Autodesk Fusion 360 part; units mm, degrees
(part 4 of 5)
  constraint parallel L69 L71
  constraint tangent L69 A64
  constraint tangent L72 A64
  constraint tangent L71 A65
  constraint tangent L72 A65
  constraint tangent L70 A66
  constraint tangent L71 A66
  constraint tangent L69 A67
  constraint tangent L70 A67
  constraint tangent L73 A68
  constraint tangent L76 A68
  constraint tangent L75 A69
  constraint tangent L76 A69
  constraint tangent L74 A70
  constraint tangent L75 A70
  constraint tangent L73 A71
  constraint tangent L74 A71
  constraint tangent L79 A72
  constraint tangent L77 A73
  constraint equal A72 A73
  constraint tangent L77 A74
  constraint tangent L78 A74
  constraint tangent L78 A75
  constraint tangent L79 A75
  constraint tangent L84 A76
  constraint tangent L85 A76
  constraint tangent L85 A77
  constraint tangent L86 A77
  constraint tangent L86 A78
  constraint tangent L87 A78
  constraint tangent L84 A79
  constraint tangent L87 A79
  constraint tangent L82 A80
  constraint tangent L83 A80
  constraint tangent L81 A81
  constraint tangent L82 A81
  constraint tangent L80 A82
  constraint tangent L81 A82
  constraint tangent L80 A83
  constraint tangent L83 A83
  constraint vertical L86
  constraint parallel L79 L86
  constraint coincident A72.start A73.end
  measures "d463" radius of A0
  measures "d464" radius of A2
  measures "d465" radius of A3
  measures "d466" radius of A6
  measures "d467" radius of A7
  measures "d468" radius of A8
  measures "d469" radius of A9
  measures "d470" radius of A10
  measures "d471" radius of A11
  measures "d472" radius of A12
  measures "d473" radius of A13
  measures "d474" radius of A14
  measures "d475" radius of A15
  measures "d476" radius of A16
  measures "d477" radius of A17
  measures "d478" radius of A18
  measures "d479" radius of A19
  measures "d480" radius of A20
  measures "d481" radius of A21
  measures "d482" radius of A22
  measures "d483" radius of A23
  measures "d484" radius of A24
  measures "d485" radius of A25
  measures "d486" radius of A26
  measures "d487" radius of A27
  measures "d488" radius of A28
  measures "d489" radius of A29
  measures "d490" radius of A30
  measures "d491" radius of A31
  measures "d492" radius of A32
  measures "d493" radius of A33
  measures "d494" radius of A34
  measures "d495" radius of A35
  measures "d496" radius of A36
  measures "d497" radius of A37
  measures "d498" radius of A38
  measures "d499" radius of A39
  measures "d500" radius of A40
  measures "d501" radius of A41
  measures "d502" radius of A42
  measures "d503" radius of A43
  measures "d504" radius of A45
  measures "d505" radius of A46
  measures "d506" radius of A47
  measures "d507" radius of A48
  measures "d508" radius of A49
  measures "d509" radius of A50
  measures "d510" radius of A51
  measures "d511" radius of A52
  measures "d512" radius of A53
  measures "d513" radius of A54
  measures "d514" radius of A55
  measures "d515" radius of A56
  measures "d516" radius of A57
  measures "d517" radius of A58
  measures "d518" radius of A59
  measures "d519" radius of A60
  measures "d520" radius of A61
  measures "d521" radius of A63
  measures "d522" radius of A64
  measures "d523" radius of A65
  measures "d524" radius of A66
  measures "d525" radius of A67
  measures "d526" radius of A68
  measures "d527" radius of A69
  measures "d528" radius of A70
  measures "d529" radius of A71
  measures "d530" radius of A72
  measures "d531" radius of A74
  measures "d532" radius of A75
  measures "d533" radius of A76
  measures "d534" radius of A77
  measures "d535" radius of A78
  measures "d536" radius of A79
  measures "d537" radius of A80
  measures "d538" radius of A81
  measures "d539" radius of A82
  measures "d540" radius of A83
extrude "Extrude10" cut sketch "Sketch22" along normal up to surface contours L7 L8 L9 A3 A4 A5 | L10 L11 L12 A6 A7 A8 | L14 L15 L16 L17 A9 A10 A11 A12 | L18 L19 L20 L21 A13 A14 A15 A16 | L23 L24 L25 L26 A17 A18 A19 A20 | L27 L28 L29 L30 A21 A22 A23 A24 | L31 L32 L33 A25 A26 A27 A28 | L34 L35 L36 A29 A30 A31 | L37 L38 L39 L40 A32 A33 A34 A35 | L41 L42 L43 A36 A37 A38 | L44 L45 L46 L47 A39 A40 A41 A42 | L48 L49 L50 A43 A44 A45 | L51 L52 L53 A46 A47 A48 | L54 L55 L56 L57 A49 A50 A51 A52 | L58 L59 L60 A53 A54 A55 | L61 L62 L63 L64 A56 A57 A58 A59 | L65 L66 L67 L68 A60 A61 A62 A63 | L69 L70 L72 A64 A65 A66 A67 | L73 L74 L75 L76 A68 A69 A70 A71 | L80 L81 L82 L83 A80 A81 A82 A83 | L84 L85 L86 L87 A76 A77 A78 A79 end surface through (-10.2751, 292.6499, 24.2874) normal (-0.992191, 0, 0.12473) offset 0
extrude "Extrude11" cut sketch "Sketch22" against normal blind 3 contours L4 L5 L6 A0 A1 A2 | L77 L78 L79 A72 A73 A74 A75
sketch "Sketch23" plane through (-113.7873, 0, 0) normal (-1, 0, 0) x (0, -1, 0)
  line L0 (-298.2923, 37.3) -> (-298, 21.0097)
  line L1 (-298, 21.0097) -> (-298.5325, 4.9975)
  line L2 (-298.5325, 4.9975) -> (-2.7182, 4.9975)
  line L3 (-2.9579, 37.3) -> (-298.2923, 37.3)
  line L4 (-3.7376, 32.7885) -> (-2.7977, 24.3512)
  line L5 (-3.3467, 19.0615) -> (-6.362, 9.8946)
  line L6 (-9.6868, 7.4883) -> (-12.9772, 7.4883)
  line L7 (-15.4767, 9.9351) -> (-15.9653, 32.9032)
  line L8 (-13.4659, 35.4563) -> (-6.7191, 35.4563)
  arc A0 (-3.7376, 32.7885) -> (-6.7191, 35.4563) centre (-6.7191, 32.4563) ccw
  arc A1 (-3.3467, 19.0615) -> (-2.7977, 24.3512) centre (-15.2208, 22.9673) ccw
  arc A2 (-9.6868, 7.4883) -> (-6.362, 9.8946) centre (-9.6868, 10.9883) ccw
  arc A3 (-15.4767, 9.9351) -> (-12.9772, 7.4883) centre (-12.9772, 9.9883) ccw
  arc A4 (-13.4659, 35.4563) -> (-15.9653, 32.9032) centre (-13.4659, 32.9563) ccw
  line L9 (-29.0847, 30.6184) -> (-17.0847, 30.6184)
  line L10 (-13.0847, 26.6184) -> (-13.0847, 14.6184)
  line L11 (-17.0847, 10.6184) -> (-29.0847, 10.6184)
  line L12 (-33.0847, 14.6184) -> (-33.0847, 26.6184)
  arc A5 (-33.0847, 14.6184) -> (-29.0847, 10.6184) centre (-29.0847, 14.6184) ccw
  arc A6 (-13.0847, 26.6184) -> (-17.0847, 30.6184) centre (-17.0847, 26.6184) ccw
  arc A7 (-17.0847, 10.6184) -> (-13.0847, 14.6184) centre (-17.0847, 14.6184) ccw
  arc A8 (-29.0847, 30.6184) -> (-33.0847, 26.6184) centre (-29.0847, 26.6184) ccw
  line L13 (-18.1072, 11.7154) -> (-18.1072, 8.9883)
  line L14 (-19.6072, 7.4883) -> (-30.6835, 7.4883)
  line L15 (-32.5016, 8.6549) -> (-32.5191, 8.693)
  line L16 (-32.0267, 10.0187) -> (-28.3251, 11.7154)
  line L17 (-28.3251, 11.7154) -> (-18.1072, 11.7154)
  arc A9 (-19.6072, 7.4883) -> (-18.1072, 8.9883) centre (-19.6072, 8.9883) ccw
  arc A10 (-32.5016, 8.6549) -> (-30.6835, 7.4883) centre (-30.6835, 9.4883) ccw
  arc A11 (-32.0267, 10.0187) -> (-32.5191, 8.693) centre (-31.61, 9.1097) ccw
  line L18 (-50.0683, 30.66) -> (-37.8488, 14.315)
  line L19 (-33.932, 14.2042) -> (-18.1542, 32.9917)
  line L20 (-19.3029, 35.4563) -> (-47.6655, 35.4563)
  arc A12 (-18.1542, 32.9917) -> (-19.3029, 35.4563) centre (-19.3029, 33.9563) ccw
  arc A13 (-47.6655, 35.4563) -> (-50.0683, 30.66) centre (-47.6655, 32.4563) ccw
  arc A14 (-37.8488, 14.315) -> (-33.932, 14.2042) centre (-35.8465, 15.812) ccw
  line L21 (-80.2589, 32.3275) -> (-72.3955, 20.8271)
  line L22 (-67.1338, 20.2294) -> (-53.4418, 32.8535)
  line L23 (-54.4585, 35.4563) -> (-78.6079, 35.4563)
  arc A15 (-53.4418, 32.8535) -> (-54.4585, 35.4563) centre (-54.4585, 33.9563) ccw
  arc A16 (-72.3955, 20.8271) -> (-67.1338, 20.2294) centre (-69.5063, 22.8025) ccw
  arc A17 (-78.6079, 35.4563) -> (-80.2589, 32.3275) centre (-78.6079, 33.4563) ccw
  line L24 (-50.8537, 28.3512) -> (-36.6087, 9.9051)
  line L25 (-37.7959, 7.4883) -> (-71.2302, 7.4883)
  line L26 (-61.4756, 22.7149) -> (-55.3137, 28.674)
  arc A18 (-50.8537, 28.3512) -> (-55.3137, 28.674) centre (-53.2281, 26.5175) ccw
  arc A19 (-37.7959, 7.4883) -> (-36.6087, 9.9051) centre (-37.7959, 8.9883) ccw
  arc A20 (-72.4665, 9.8377) -> (-71.2302, 7.4883) centre (-71.2302, 8.9883) ccw
  arc A21 (-61.4756, 22.7149) -> (-72.5137, 9.7645) centre (0.0474, -40.9024) ccw
  line L27 (-82.205, 31.3656) -> (-72.5578, 17.4373)
  line L28 (-72.8035, 13.7118) -> (-73.5988, 12.8364)
  line L29 (-78.0703, 11.8224) -> (-104.2986, 22.522)
  line L30 (-105.4935, 24.8169) -> (-103.8723, 31.9532)
  line L31 (-99.4841, 35.4563) -> (-90.0147, 35.4563)
  arc A22 (-78.0703, 11.8224) -> (-73.5988, 12.8364) centre (-76.5594, 15.5261) ccw
  arc A23 (-72.8035, 13.7118) -> (-72.5578, 17.4373) centre (-75.024, 15.7291) ccw
  arc A24 (-82.205, 31.3656) -> (-90.0147, 35.4563) centre (-90.0147, 25.9563) ccw
  arc A25 (-99.4841, 35.4563) -> (-103.8723, 31.9532) centre (-99.4841, 30.9563) ccw
  arc A26 (-105.4935, 24.8169) -> (-104.2986, 22.522) centre (-103.5432, 24.3738) ccw
  line L32 (-102.0259, 19.6707) -> (-78.925, 9.4021)
  line L33 (-79.3311, 7.4883) -> (-116.1348, 7.4883)
  line L34 (-117.4703, 10.977) -> (-109.0066, 18.5695)
  arc A27 (-102.0259, 19.6707) -> (-109.0066, 18.5695) centre (-104.6662, 13.7311) ccw
  arc A28 (-79.3311, 7.4883) -> (-78.925, 9.4021) centre (-79.3311, 8.4883) ccw
  arc A29 (-117.4703, 10.977) -> (-116.1348, 7.4883) centre (-116.1348, 9.4883) ccw
  line L35 (-127.6369, 31.7266) -> (-123.0407, 13.3976)
  line L36 (-118.0109, 12.0045) -> (-109.066, 20.9374)
  line L37 (-106.5273, 25.9576) -> (-105.6108, 32.007)
  line L38 (-108.577, 35.4563) -> (-124.727, 35.4563)
  arc A30 (-105.6108, 32.007) -> (-108.577, 35.4563) centre (-108.577, 32.4563) ccw
  arc A31 (-109.066, 20.9374) -> (-106.5273, 25.9576) centre (-115.4257, 27.3056) ccw
  arc A32 (-123.0407, 13.3976) -> (-118.0109, 12.0045) centre (-120.1308, 14.1272) ccw
  arc A33 (-124.727, 35.4563) -> (-127.6369, 31.7266) centre (-124.727, 32.4563) ccw
  line L39 (-130.3627, 33.6384) -> (-123.8711, 10.6682)
  line L40 (-126.2769, 7.4883) -> (-169.5459, 7.4883)
  line L41 (-170.2607, 9.1876) -> (-147.4375, 32.5152)
  line L42 (-139.5747, 35.8225) -> (-133.2496, 35.8225)
  arc A34 (-130.3627, 33.6384) -> (-133.2496, 35.8225) centre (-133.2496, 32.8225) ccw
  arc A35 (-139.5747, 35.8225) -> (-147.4375, 32.5152) centre (-139.5747, 24.8225) ccw
  arc A36 (-126.2769, 7.4883) -> (-123.8711, 10.6682) centre (-126.2769, 9.9883) ccw
  arc A37 (-170.2607, 9.1876) -> (-169.5459, 7.4883) centre (-169.5459, 8.4883) ccw
  line L43 (-171.6146, 10.8227) -> (-150.4805, 32.4238)
  line L44 (-151.9101, 35.8225) -> (-177.6214, 35.8225)
  line L45 (-181.99, 32.4024) -> (-182.3695, 30.8671)
  line L46 (-181.8959, 26.7134) -> (-174.0246, 11.1932)
  arc A38 (-182.3695, 30.8671) -> (-181.8959, 26.7134) centre (-176.5448, 29.4273) ccw
  arc A39 (-177.6214, 35.8225) -> (-181.99, 32.4024) centre (-177.6214, 31.3225) ccw
  arc A40 (-174.0246, 11.1932) -> (-171.6146, 10.8227) centre (-172.6868, 11.8717) ccw
  arc A41 (-150.4805, 32.4238) -> (-151.9101, 35.8225) centre (-151.9101, 33.8225) ccw
  line L47 (-182.5845, 22.9873) -> (-176.1226, 9.642)
  line L48 (-177.4726, 7.4883) -> (-194.767, 7.4883)
  line L49 (-198.7537, 11.8145) -> (-197.7367, 24.2445)
  line L50 (-194.1507, 26.9401) -> (-185.39, 25.1643)
  line L51 (-196.251, 35.416) -> (-188.0937, 35.416)
  line L52 (-184.719, 32.844) -> (-184.0663, 30.4707)
  line L53 (-186.392, 27.9802) -> (-195.9523, 29.9181)
  line L54 (-198.7566, 33.2991) -> (-198.7508, 32.8808)
  arc A42 (-196.251, 35.416) -> (-198.7508, 32.8808) centre (-196.251, 32.916) ccw
  arc A43 (-198.7566, 33.2991) -> (-195.9523, 29.9181) centre (-195.257, 33.3483) ccw
  arc A44 (-184.719, 32.844) -> (-188.0937, 35.416) centre (-188.0937, 31.916) ccw
  arc A45 (-186.392, 27.9802) -> (-184.0663, 30.4707) centre (-185.9947, 29.9403) ccw
  arc A46 (-182.5845, 22.9873) -> (-185.39, 25.1643) centre (-186.1846, 21.244) ccw
  arc A47 (-194.1507, 26.9401) -> (-197.7367, 24.2445) centre (-194.7467, 23.9999) ccw
  arc A48 (-198.7537, 11.8145) -> (-194.767, 7.4883) centre (-194.767, 11.4883) ccw
  arc A49 (-177.4726, 7.4883) -> (-176.1226, 9.642) centre (-177.4726, 8.9883) ccw
  line L55 (-201.3181, 31.0173) -> (-201.8048, 31.4581)
  line L56 (-206.287, 30.9396) -> (-212.4198, 22.0615)
  line L57 (-212.1436, 17.1592) -> (-204.0082, 7.8292)
  line L58 (-200.5039, 9.0318) -> (-199.5188, 26.6333)
  arc A50 (-212.4198, 22.0615) -> (-212.1436, 17.1592) centre (-209.1287, 19.7881) ccw
  arc A51 (-204.0082, 7.8292) -> (-200.5039, 9.0318) centre (-202.5008, 9.1436) ccw
  arc A52 (-201.8048, 31.4581) -> (-206.287, 30.9396) centre (-203.8187, 29.2345) ccw
  arc A53 (-199.5188, 26.6333) -> (-201.3181, 31.0173) centre (-205.0102, 26.9407) ccw
  line L59 (-228.1983, 31.0611) -> (-217.2747, 25.9128)
  line L60 (-213.7346, 26.655) -> (-208.6312, 32.5081)
  line L61 (-210.1386, 35.8225) -> (-227.1325, 35.8225)
  arc A54 (-227.1325, 35.8225) -> (-228.1983, 31.0611) centre (-227.1325, 33.3225) ccw
  arc A55 (-208.6312, 32.5081) -> (-210.1386, 35.8225) centre (-210.1386, 33.8225) ccw
  arc A56 (-217.2747, 25.9128) -> (-213.7346, 26.655) centre (-215.9958, 28.6265) ccw
  line L62 (-225.5242, 26.6005) -> (-216.6046, 22.0447)
  line L63 (-216.798, 17.5033) -> (-226.1871, 13.6752)
  line L64 (-230.2345, 14.721) -> (-234.2485, 19.7054)
  line L65 (-234.2168, 22.88) -> (-232.2401, 25.2369)
  arc A57 (-225.5242, 26.6005) -> (-232.2401, 25.2369) centre (-228.026, 21.7025) ccw
  arc A58 (-234.2168, 22.88) -> (-234.2485, 19.7054) centre (-232.3013, 21.2734) ccw
  arc A59 (-230.2345, 14.721) -> (-226.1871, 13.6752) centre (-227.5085, 16.9162) ccw
  arc A60 (-216.798, 17.5033) -> (-216.6046, 22.0447) centre (-217.7418, 19.8183) ccw
  line L66 (-212.773, 14.8416) -> (-208.1185, 10.0313)
  line L67 (-209.1965, 7.4883) -> (-221.7705, 7.4883)
  line L68 (-225.0064, 11.8674) -> (-216.7262, 15.5987)
  arc A61 (-225.7961, 9.9772) -> (-221.7705, 7.4883) centre (-221.7705, 11.9883) ccw
  arc A62 (-225.0064, 11.8674) -> (-225.7961, 9.9772) centre (-224.3901, 10.4998) ccw
  arc A63 (-212.773, 14.8416) -> (-216.7262, 15.5987) centre (-215.2883, 12.4077) ccw
  arc A64 (-209.1965, 7.4883) -> (-208.1185, 10.0313) centre (-209.1965, 8.9883) ccw
  line L69 (-243.5581, 13.7607) -> (-238.5407, 7.9849)
  line L70 (-235.3648, 8.1899) -> (-232.5294, 12.459)
  line L71 (-232.7955, 14.9938) -> (-235.9763, 18.1116)
  line L72 (-239.6311, 19.1626) -> (-241.9344, 18.6588)
  arc A65 (-235.9763, 18.1116) -> (-239.6311, 19.1626) centre (-238.7763, 15.255) ccw
  arc A66 (-241.9344, 18.6588) -> (-243.5581, 13.7607) centre (-241.2933, 15.7281) ccw
  arc A67 (-232.5294, 12.459) -> (-232.7955, 14.9938) centre (-234.1955, 13.5655) ccw
  arc A68 (-238.5407, 7.9849) -> (-235.3648, 8.1899) centre (-237.0309, 9.2965) ccw
  line L73 (-240.9685, 21.1417) -> (-236.0861, 22.7103)
  line L74 (-234.8254, 23.9119) -> (-232.4395, 30.2703)
  line L75 (-234.1781, 35.8225) -> (-262.6295, 35.8225)
  line L76 (-263.938, 31.1923) -> (-248.9657, 21.9955)
  line L77 (-246.7988, 21.2283) -> (-244.0157, 20.865)
  arc A69 (-236.0861, 22.7103) -> (-234.8254, 23.9119) centre (-236.6979, 24.6145) ccw
  arc A70 (-244.0157, 20.865) -> (-240.9685, 21.1417) centre (-243.1097, 27.8062) ccw
  arc A71 (-248.9657, 21.9955) -> (-246.7988, 21.2283) centre (-246.087, 26.682) ccw
  arc A72 (-262.6295, 35.8225) -> (-263.938, 31.1923) centre (-262.6295, 33.3225) ccw
  line L78 (-233.2969, 35.2953) -> (-232.701, 34.1846)
  arc A73 (-233.2969, 35.2953) -> (-234.1781, 35.8225) centre (-234.1781, 34.8225) ccw
  arc A74 (-232.4395, 30.2703) -> (-232.701, 34.1846) centre (-236.8867, 31.939) ccw
  line L79 (-264.8466, 28.7558) -> (-247.5589, 17.5714)
  line L80 (-247.3226, 14.392) -> (-249.8693, 12.1467)
  line L81 (-253.9757, 12.2768) -> (-267.3479, 25.6631)
  arc A75 (-264.8466, 28.7558) -> (-267.3479, 25.6631) centre (-265.9329, 27.0765) ccw
  arc A76 (-253.9757, 12.2768) -> (-249.8693, 12.1467) centre (-251.8532, 14.397) ccw
  arc A77 (-247.3226, 14.392) -> (-247.5589, 17.5714) centre (-248.6453, 15.8922) ccw
  line L82 (-291.141, 35.5263) -> (-293.8507, 35.1983)
  line L83 (-296.4896, 32.1574) -> (-296.3543, 25.6768)
  line L84 (-284.738, 23.6942) -> (-282.7176, 29.0788)
  line L85 (-284.2734, 32.8585) -> (-289.5274, 35.2738)
  arc A78 (-289.5274, 35.2738) -> (-291.141, 35.5263) centre (-290.7805, 32.548) ccw
  arc A79 (-282.7176, 29.0788) -> (-284.2734, 32.8585) centre (-285.5264, 30.1327) ccw
  arc A80 (-296.3543, 25.6768) -> (-284.738, 23.6942) centre (-290.3556, 25.802) ccw
  arc A81 (-293.8507, 35.1983) -> (-296.4896, 32.1574) centre (-293.4902, 32.2201) ccw
  line L86 (-295.786, 17.2442) -> (-295.3907, 10.7748)
  line L87 (-291.8972, 7.4883) -> (-280.6831, 7.4883)
  line L88 (-279.7034, 10.1242) -> (-281.7456, 11.8854)
  line L89 (-284.5387, 13.805) -> (-293.5794, 18.6573)
  arc A82 (-293.5794, 18.6573) -> (-295.786, 17.2442) centre (-294.2888, 17.3357) ccw
  arc A83 (-281.7456, 11.8854) -> (-284.5387, 13.805) centre (-291.8687, 0.1478) ccw
  arc A84 (-280.6831, 7.4883) -> (-279.7034, 10.1242) centre (-280.6831, 8.9883) ccw
  arc A85 (-295.3907, 10.7748) -> (-291.8972, 7.4883) centre (-291.8972, 10.9883) ccw
  line L90 (-267.8373, 31.4338) -> (-275.7739, 16.2362)
  line L91 (-281.8887, 15.022) -> (-282.1098, 15.2072)
  line L92 (-283.8736, 21.9137) -> (-279.385, 33.8764)
  line L93 (-276.5762, 35.8225) -> (-270.4965, 35.8225)
  arc A86 (-276.5762, 35.8225) -> (-279.385, 33.8764) centre (-276.5762, 32.8225) ccw
  arc A87 (-267.8373, 31.4338) -> (-270.4965, 35.8225) centre (-270.4965, 32.8225) ccw
  arc A88 (-281.8887, 15.022) -> (-275.7739, 16.2362) centre (-279.3195, 18.0878) ccw
  arc A89 (-283.8736, 21.9137) -> (-282.1098, 15.2072) centre (-278.256, 19.8059) ccw
  line L94 (-266.8843, 20.7953) -> (-256.1487, 10.0484)
  line L95 (-257.2099, 7.4883) -> (-273.466, 7.4883)
  line L96 (-275.2388, 10.4141) -> (-270.0721, 20.3076)
  arc A90 (-266.8843, 20.7953) -> (-270.0721, 20.3076) centre (-268.2993, 19.3818) ccw
  arc A91 (-275.2388, 10.4141) -> (-273.466, 7.4883) centre (-273.466, 9.4883) ccw
  arc A92 (-257.2099, 7.4883) -> (-256.1487, 10.0484) centre (-257.2099, 8.9883) ccw
  line L97 (-2.7182, 4.9975) -> (-3.2504, 21.0001)
  line L98 (-3.2504, 21.0001) -> (-2.9579, 37.3)
  point P0 (-33.0847, 30.6184)
  point P1 (-13.0847, 30.6184)
  point P2 (-33.0847, 10.6184)
  dimension "d545" = 3
  dimension "d546" = 12.5
  dimension "d547" = 3.5
  dimension "d548" = 2.5
  dimension "d549" = 2.5
  dimension "d550" = 20
  dimension "d551" = 20
  dimension "d552" = 4
  dimension "d553" = 1.5
  dimension "d554" = 2
  dimension "d555" = 1
  dimension "d556" = 1.5
  dimension "d557" = 3
  dimension "d558" = 2.5
  dimension "d559" = 1.5
  dimension "d560" = 3.5
  dimension "d561" = 2
  dimension "d562" = 3
  dimension "d563" = 1.5
  dimension "d564" = 1.5
  dimension "d565" = 88.5
  dimension "d566" = 4
  dimension "d567" = 3
  dimension "d568" = 9.5
  dimension "d569" = 4.5
  dimension "d570" = 2
  dimension "d571" = 6.5
  dimension "d572" = 1
  dimension "d573" = 2
  dimension "d574" = 3
  dimension "d575" = 9
  dimension "d576" = 3
  dimension "d577" = 3
  dimension "d578" = 3
  dimension "d579" = 11
  dimension "d580" = 2.5
  dimension "d581" = 1
  dimension "d582" = 6
  dimension "d583" = 4.5
  dimension "d584" = 1.5
  dimension "d585" = 2
  dimension "d586" = 2.5
  dimension "d587" = 3.5
  dimension "d588" = 3.5
  dimension "d589" = 2
  dimension "d590" = 4
  dimension "d591" = 3
  dimension "d592" = 4
  dimension "d593" = 1.5
  dimension "d594" = 4
  dimension "d595" = 2
  dimension "d596" = 3
  dimension "d597" = 5.5
  dimension "d598" = 2.5
  dimension "d599" = 2
  dimension "d600" = 3
  dimension "d601" = 5.5
  dimension "d602" = 2.5
  dimension "d603" = 3.5
  dimension "d604" = 2.5
  dimension "d605" = 4.5
  dimension "d606" = 1.5
  dimension "d607" = 3.5
  dimension "d608" = 1.5
  dimension "d609" = 4
  dimension "d610" = 3
  dimension "d611" = 2
  dimension "d612" = 2
  dimension "d615" = 2
  dimension "d616" = 7
  dimension "d617" = 5.5
  dimension "d618" = 2.5
  dimension "d619" = 1
  dimension "d620" = 4.75
  dimension "d621" = 2
  dimension "d622" = 3
  dimension "d623" = 2
  dimension "d624" = 3
  dimension "d625" = 3
  dimension "d626" = 6
  dimension "d627" = 3
  dimension "d628" = 1.5
  dimension "d629" = 15.5
  dimension "d630" = 1.5
  dimension "d631" = 3.5
  dimension "d632" = 3
  dimension "d633" = 3
  dimension "d634" = 4
  dimension "d635" = 6
  dimension "d636" = 2
  dimension "d637" = 2
  dimension "d638" = 1.5
  constraint horizontal L6
  constraint horizontal L8
  constraint tangent L4 A0
  constraint tangent L8 A0
  constraint tangent L4 A1
  constraint tangent L5 A1
  constraint tangent L5 A2
  constraint tangent L6 A2
  constraint tangent L6 A3
  constraint tangent L7 A3
  constraint tangent L7 A4
  constraint tangent L8 A4
  constraint horizontal L9
  constraint vertical L10
  constraint horizontal L11
  constraint vertical L12
  constraint coincident P2 L11
  constraint coincident P2 L12
  constraint tangent L11 A5
  constraint tangent L12 A5
  constraint coincident P1 L9
  constraint coincident P1 L10
  constraint tangent L9 A6
  constraint tangent L10 A6
  constraint equal A5 A6
  constraint tangent L10 A7
  constraint tangent L11 A7
  constraint equal A5 A7
  constraint coincident P0 L9
  constraint coincident P0 L12
  constraint tangent L9 A8
  constraint tangent L12 A8
  constraint equal A5 A8
  constraint perpendicular L11 L13
  constraint perpendicular L13 L14
  constraint perpendicular L15 L16
  constraint perpendicular L13 L17
  constraint tangent L13 A9
  constraint tangent L14 A9
  constraint tangent L14 A10
  constraint tangent L15 A10
  constraint tangent L15 A11
  constraint tangent L16 A11
  constraint horizontal L20
  constraint collinear L8 L20
  constraint tangent L19 A12
  constraint tangent L20 A12
  constraint tangent L18 A13
  constraint tangent L20 A13
  constraint tangent L18 A14
  constraint tangent L19 A14
  constraint horizontal L23
  constraint collinear L20 L23
  constraint tangent L22 A15
  constraint tangent L23 A15
  constraint tangent L21 A16
  constraint tangent L22 A16
  constraint tangent L21 A17
  constraint tangent L23 A17
  constraint horizontal L25
  constraint tangent L24 A18
  constraint tangent L26 A18
  constraint tangent L24 A19
  constraint tangent L25 A19
  constraint tangent L25 A20
  constraint tangent L26 A21
  constraint horizontal L31
  constraint collinear L23 L31
  constraint tangent L28 A22
  constraint tangent L29 A22
  constraint tangent L27 A23
  constraint tangent L28 A23
  constraint tangent L27 A24
  constraint tangent L31 A24
  constraint tangent L30 A25
  constraint tangent L31 A25
  constraint tangent L29 A26
  constraint tangent L30 A26
  constraint coincident A20 A21.end
  constraint horizontal L33
  constraint collinear L6 L14
  constraint collinear L14 L25
  constraint collinear L25 L33
  constraint tangent L32 A27
  constraint tangent L34 A27
  constraint tangent L32 A28
  constraint tangent L33 A28
  constraint tangent L33 A29
  constraint tangent L34 A29
  constraint horizontal L38
  constraint collinear L31 L38
  constraint tangent L37 A30
  constraint tangent L38 A30
  constraint tangent L36 A31
  constraint tangent L37 A31
  constraint tangent L35 A32
  constraint tangent L36 A32
  constraint tangent L35 A33
  constraint tangent L38 A33
  constraint horizontal L40
  constraint horizontal L42
  constraint collinear L33 L40
  constraint tangent L39 A34
  constraint tangent L42 A34
  constraint tangent L41 A35
  constraint tangent L42 A35
  constraint tangent L39 A36
  constraint tangent L40 A36
  constraint tangent L41 A37
  constraint tangent L40 A37
  constraint parallel L41 L43
  constraint parallel L2 L44
  constraint tangent L45 A38
  constraint tangent L46 A38
  constraint tangent L44 A39
  constraint tangent L45 A39
  constraint tangent L43 A40
  constraint tangent L46 A40
  constraint tangent L43 A41
  constraint tangent L44 A41
  constraint collinear L42 L44
  constraint horizontal L48
  constraint parallel L50 L53
  constraint tangent L51 A42
  constraint tangent L54 A42
  constraint tangent L53 A43
  constraint tangent L54 A43
  constraint tangent L51 A44
  constraint tangent L52 A44
  constraint tangent L52 A45
  constraint tangent L53 A45
  constraint tangent L47 A46
  constraint tangent L50 A46
  constraint tangent L49 A47
  constraint tangent L50 A47
  constraint tangent L48 A48
  constraint tangent L49 A48
  constraint tangent L47 A49
  constraint tangent L48 A49
  constraint collinear L40 L48
  constraint tangent L56 A50
  constraint tangent L57 A50
  constraint tangent L57 A51
  constraint tangent L58 A51
  constraint tangent L55 A52
  constraint tangent L56 A52
  constraint tangent L55 A53
  constraint tangent L58 A53
  constraint tangent L61 A54
  constraint tangent L59 A54
  constraint tangent L60 A55
  constraint tangent L61 A55
  constraint tangent L59 A56
  constraint tangent L60 A56
  constraint horizontal L61
  constraint collinear L44 L61
  constraint horizontal L51
  constraint tangent L62 A57
  constraint tangent L65 A57
  constraint tangent L64 A58
  constraint tangent L65 A58
  constraint tangent L63 A59
  constraint tangent L64 A59
  constraint tangent L62 A60
  constraint tangent L63 A60
  constraint horizontal L67
  constraint collinear L48 L67
  constraint tangent L67 A61
  constraint tangent L68 A62
  constraint coincident A61.start A62.end
  constraint tangent L68 A63
  constraint tangent L66 A63
  constraint tangent L66 A64
  constraint tangent L67 A64
  constraint tangent L71 A65
  constraint tangent L72 A65
  constraint tangent L69 A66
  constraint tangent L72 A66
  constraint tangent L70 A67
  constraint tangent L71 A67
  constraint tangent L69 A68
  constraint tangent L70 A68
  constraint horizontal L75
  constraint collinear L61 L75
  constraint tangent L73 A69
  constraint tangent L74 A69
  constraint tangent L73 A70
  constraint tangent L77 A70
  constraint tangent L76 A71
  constraint tangent L77 A71
  constraint tangent L75 A72
  constraint tangent L76 A72
  constraint tangent L75 A73
  constraint tangent L78 A73
  constraint tangent L74 A74
  constraint tangent L78 A74
  constraint tangent L81 A75
  constraint tangent L79 A75
  constraint tangent L80 A76
  constraint tangent L81 A76
  constraint tangent L79 A77
  constraint tangent L80 A77
  constraint tangent L82 A78
  constraint tangent L85 A78
  constraint tangent L84 A79
  constraint tangent L85 A79
  constraint tangent L83 A80
  constraint tangent L84 A80
  constraint tangent L82 A81
  constraint tangent L83 A81
  constraint horizontal L87
  constraint tangent L86 A82
  constraint tangent L89 A82
  constraint tangent L88 A83
  constraint tangent L89 A83
  constraint tangent L87 A84
  constraint tangent L88 A84
  constraint tangent L86 A85
  constraint tangent L87 A85
  constraint horizontal L93
  constraint collinear L75 L93
  constraint tangent L92 A86
  constraint tangent L93 A86
  constraint tangent L90 A87
  constraint tangent L93 A87
  constraint tangent L90 A88
  constraint tangent L91 A88
  constraint tangent L91 A89
  constraint tangent L92 A89
  constraint parallel L84 L92
  constraint horizontal L95
  constraint collinear L67 L95
  constraint collinear L87 L95
  constraint tangent L94 A90
  constraint tangent L96 A90
  constraint tangent L95 A91
  constraint tangent L96 A91
  constraint tangent L94 A92
  constraint tangent L95 A92
  constraint parallel L90 L96
  constraint parallel L81 L94
  measures "d545" radius of A0
  measures "d546" radius of A1
  measures "d547" radius of A2
  measures "d548" radius of A3
  measures "d549" radius of A4
  measures "d550" distance of P0 P1
  measures "d551" distance of P0 P2
  measures "d552" radius of A5
  measures "d553" radius of A9
  measures "d554" radius of A10
  measures "d555" radius of A11
  measures "d556" radius of A12
  measures "d557" radius of A13
  measures "d558" radius of A14
  measures "d559" radius of A15
  measures "d560" radius of A16
  measures "d561" radius of A17
  measures "d562" radius of A18
  measures "d563" radius of A19
  measures "d564" radius of A20
  measures "d565" radius of A21
  measures "d566" radius of A22
  measures "d567" radius of A23
  measures "d568" radius of A24
  measures "d569" radius of A25
  measures "d570" radius of A26
  measures "d571" radius of A27
  measures "d572" radius of A28
  measures "d573" radius of A29
  measures "d574" radius of A30
  measures "d575" radius of A31
  measures "d576" radius of A32
  measures "d577" radius of A33
  measures "d578" radius of A34
  measures "d579" radius of A35
  measures "d580" radius of A36
  measures "d581" radius of A37
  measures "d582" radius of A38
  measures "d583" radius of A39
  measures "d584" radius of A40
  measures "d585" radius of A41
  measures "d586" radius of A42
  measures "d587" radius of A43
  measures "d588" radius of A44
  measures "d589" radius of A45
  measures "d590" radius of A46
  measures "d591" radius of A47
  measures "d592" radius of A48
  measures "d593" radius of A49
  measures "d594" radius of A50
  measures "d595" radius of A51
  measures "d596" radius of A52
  measures "d597" radius of A53
  measures "d598" radius of A54
  measures "d599" radius of A55
  measures "d600" radius of A56
  measures "d601" radius of A57
  measures "d602" radius of A58
  measures "d603" radius of A59
  measures "d604" radius of A60
  measures "d605" radius of A61
  measures "d606" radius of A62
  measures "d607" radius of A63
  measures "d608" radius of A64
  measures "d609" radius of A65
  measures "d610" radius of A66
  measures "d611" radius of A67
  measures "d612" radius of A68
  measures "d615" radius of A69
  measures "d616" radius of A70
  measures "d617" radius of A71
  measures "d618" radius of A72
  measures "d619" radius of A73
  measures "d620" radius of A74
  measures "d621" radius of A75
  measures "d622" radius of A76
  measures "d623" radius of A77
  measures "d624" radius of A78
  measures "d625" radius of A79
  measures "d626" radius of A80
  measures "d627" radius of A81
  measures "d628" radius of A82
  measures "d629" radius of A83
  measures "d630" radius of A84
  measures "d631" radius of A85
  measures "d632" radius of A86
  measures "d633" radius of A87
  measures "d634" radius of A88
  measures "d635" radius of A89
  measures "d636" radius of A90
  measures "d637" radius of A91
  measures "d638" radius of A92
ref_plane "WorkPlane10" through (-109.4382, 7.3501, 19.6195) normal (-0.992191, 0, 0.12473) x (0, -1, 0)
extrude "Extrude12" cut sketch "Sketch23" along normal up to surface contours L9 L12 A8 L18 L19 L20 A12 A13 A14 | L11 A5 L13 L14 L15 L16 A9 A10 A11 | L21 L22 L23 A15 A16 A17 | L24 L25 L26 A18 A19 A20 A21 | L27 L28 L29 L30 L31 A22 A23 A24 A25 A26 | L32 L33 L34 A27 A28 A29 | L35 L36 L37 L38 A30 A31 A32 A33 | L39 L40 L41 L42 A34 A35 A36 A37 | L43 L44 L45 L46 A38 A39 A40 A41 | L47 L48 L49 L50 A46 A47 A48 A49 | L51 L52 L53 A42 A43 A44 A45 | L55 L56 L57 L58 A50 A51 A52 A53 | L59 L60 L61 A54 A55 A56 | L62 L63 L64 L65 A57 A58 A59 A60 | L66 L67 L68 A61 A62 A63 A64 | L69 L70 L71 L72 A65 A66 A67 A68 | L73 L74 L75 L76 L77 A69 A70 A71 A72 L78 A73 A74 | L79 L80 L81 A75 A76 A77 | L90 L91 L92 L93 A86 A87 A88 A89 | L94 L95 L96 A90 A91 A92 end surface through (-109.4382, 7.3501, 19.6195) normal (-0.992191, 0, 0.12473) offset 0
extrude "Extrude13" cut sketch "Sketch23" against normal blind 4 contours L4 L5 L6 L7 L8 A0 A1 A2 A3 A4 L10 A6 A7 L97 L98 | L4 A1 L97 L98 | L82 L83 L84 L85 A78 A79 A80 A81 | L86 L87 L88 L89 A82 A83 A84 A85
sketch "Sketch24" plane through (-113.7873, 0, 0) normal (-1, 0, 0) x (0, -1, 0)
  line L0 (-3.3467, 19.0615) -> (-6.362, 9.8946)
  arc A0 (-9.6868, 7.4883) -> (-6.362, 9.8946) centre (-9.6868, 10.9883) ccw
  line L1 (-9.6868, 7.4883) -> (-12.9772, 7.4883)
  arc A1 (-15.4767, 9.9351) -> (-12.9772, 7.4883) centre (-12.9772, 9.9883) ccw
  line L2 (-15.4767, 9.9351) -> (-15.4982, 10.9465)
  arc A2 (-15.4982, 10.9465) -> (-13.0847, 14.6184) centre (-17.0847, 14.6184) ccw
  line L3 (-13.0847, 14.6184) -> (-13.0847, 26.6184)
  arc A3 (-13.0847, 26.6184) -> (-15.913, 30.4429) centre (-17.0847, 26.6184) ccw
  line L4 (-15.913, 30.4429) -> (-15.9653, 32.9032)
  arc A4 (-13.4659, 35.4563) -> (-15.9653, 32.9032) centre (-13.4659, 32.9563) ccw
  line L5 (-13.4659, 35.4563) -> (-6.7191, 35.4563)
  arc A5 (-3.7376, 32.7885) -> (-6.7191, 35.4563) centre (-6.7191, 32.4563) ccw
  line L6 (-280.6831, 7.4883) -> (-291.8972, 7.4883)
  arc A6 (-295.3907, 10.7748) -> (-291.8972, 7.4883) centre (-291.8972, 10.9883) ccw
  line L7 (-293.5794, 18.6573) -> (-284.5387, 13.805)
  arc A7 (-281.7456, 11.8854) -> (-284.5387, 13.805) centre (-291.8687, 0.1478) ccw
  line L8 (-281.7456, 11.8854) -> (-279.7034, 10.1242)
  arc A8 (-280.6831, 7.4883) -> (-279.7034, 10.1242) centre (-280.6831, 8.9883) ccw
  line L9 (-296.3543, 25.6768) -> (-296.4896, 32.1574)
  arc A9 (-289.5274, 35.2738) -> (-291.141, 35.5263) centre (-290.7805, 32.548) ccw
  line L10 (-289.5274, 35.2738) -> (-284.2734, 32.8585)
  arc A10 (-282.7176, 29.0788) -> (-284.2734, 32.8585) centre (-285.5264, 30.1327) ccw
  line L11 (-282.7176, 29.0788) -> (-284.738, 23.6942)
  arc A11 (-296.3543, 25.6768) -> (-284.738, 23.6942) centre (-290.3556, 25.802) ccw
  line L12 (-253.9757, 12.2768) -> (-267.3479, 25.6631)
  arc A12 (-264.8466, 28.7558) -> (-267.3479, 25.6631) centre (-265.9329, 27.0765) ccw
  line L13 (-264.8466, 28.7558) -> (-247.5589, 17.5714)
  arc A13 (-247.3226, 14.392) -> (-247.5589, 17.5714) centre (-248.6453, 15.8922) ccw
  line L14 (-247.3226, 14.392) -> (-249.8693, 12.1467)
  arc A14 (-253.9757, 12.2768) -> (-249.8693, 12.1467) centre (-251.8532, 14.397) ccw
  arc A15 (-234.2168, 22.88) -> (-234.2485, 19.7054) centre (-232.3013, 21.2734) ccw
  line L15 (-234.2168, 22.88) -> (-232.2401, 25.2369)
  arc A16 (-225.5242, 26.6005) -> (-232.2401, 25.2369) centre (-228.026, 21.7025) ccw
  line L16 (-225.5242, 26.6005) -> (-216.6046, 22.0447)
  arc A17 (-216.798, 17.5033) -> (-216.6046, 22.0447) centre (-217.7418, 19.8183) ccw
  line L17 (-216.798, 17.5033) -> (-226.1871, 13.6752)
  arc A18 (-230.2345, 14.721) -> (-226.1871, 13.6752) centre (-227.5085, 16.9162) ccw
  line L18 (-230.2345, 14.721) -> (-234.2485, 19.7054)
  arc A19 (-194.1507, 26.9401) -> (-197.7367, 24.2445) centre (-194.7467, 23.9999) ccw
  line L19 (-194.1507, 26.9401) -> (-185.39, 25.1643)
  arc A20 (-182.5845, 22.9873) -> (-185.39, 25.1643) centre (-186.1846, 21.244) ccw
  line L20 (-182.5845, 22.9873) -> (-176.1226, 9.642)
  arc A21 (-177.4726, 7.4883) -> (-176.1226, 9.642) centre (-177.4726, 8.9883) ccw
  line L21 (-177.4726, 7.4883) -> (-194.767, 7.4883)
  arc A22 (-198.7537, 11.8145) -> (-194.767, 7.4883) centre (-194.767, 11.4883) ccw
  line L22 (-198.7537, 11.8145) -> (-197.7367, 24.2445)
  line L23 (-102.0259, 19.6707) -> (-78.925, 9.4021)
  arc A23 (-79.3311, 7.4883) -> (-78.925, 9.4021) centre (-79.3311, 8.4883) ccw
  line L24 (-79.3311, 7.4883) -> (-116.1348, 7.4883)
  arc A24 (-117.4703, 10.977) -> (-116.1348, 7.4883) centre (-116.1348, 9.4883) ccw
  line L25 (-117.4703, 10.977) -> (-109.0066, 18.5695)
  arc A25 (-102.0259, 19.6707) -> (-109.0066, 18.5695) centre (-104.6662, 13.7311) ccw
  line L26 (-18.1072, 10.6184) -> (-18.1072, 8.9883)
  arc A26 (-19.6072, 7.4883) -> (-18.1072, 8.9883) centre (-19.6072, 8.9883) ccw
  line L27 (-19.6072, 7.4883) -> (-30.6835, 7.4883)
  arc A27 (-32.5016, 8.6549) -> (-30.6835, 7.4883) centre (-30.6835, 9.4883) ccw
  line L28 (-32.5016, 8.6549) -> (-32.5191, 8.693)
  arc A28 (-32.0267, 10.0187) -> (-32.5191, 8.693) centre (-31.61, 9.1097) ccw
  line L29 (-32.0267, 10.0187) -> (-30.3035, 10.8086)
  arc A29 (-30.3035, 10.8086) -> (-29.0847, 10.6184) centre (-29.0847, 14.6184) ccw
  line L30 (-29.0847, 10.6184) -> (-18.1072, 10.6184)
  arc A30 (-37.7959, 7.4883) -> (-36.6087, 9.9051) centre (-37.7959, 8.9883) ccw
  line L31 (-37.7959, 7.4883) -> (-71.2302, 7.4883)
  arc A31 (-72.5137, 9.7645) -> (-71.2302, 7.4883) centre (-71.2302, 8.9883) ccw
  arc A32 (-61.4756, 22.7149) -> (-72.5137, 9.7645) centre (0.0474, -40.9024) ccw
  line L32 (-61.4756, 22.7149) -> (-55.3137, 28.674)
  arc A33 (-50.8537, 28.3512) -> (-55.3137, 28.674) centre (-53.2281, 26.5175) ccw
  line L33 (-50.8537, 28.3512) -> (-36.6087, 9.9051)
  arc A34 (-105.6108, 32.007) -> (-108.577, 35.4563) centre (-108.577, 32.4563) ccw
  line L34 (-105.6108, 32.007) -> (-106.5273, 25.9576)
  arc A35 (-109.066, 20.9374) -> (-106.5273, 25.9576) centre (-115.4257, 27.3056) ccw
  line L35 (-109.066, 20.9374) -> (-118.0109, 12.0045)
  arc A36 (-123.0407, 13.3976) -> (-118.0109, 12.0045) centre (-120.1308, 14.1272) ccw
  line L36 (-123.0407, 13.3976) -> (-127.6369, 31.7266)
  arc A37 (-124.727, 35.4563) -> (-127.6369, 31.7266) centre (-124.727, 32.4563) ccw
  line L37 (-124.727, 35.4563) -> (-108.577, 35.4563)
  arc A38 (-184.719, 32.844) -> (-188.0937, 35.416) centre (-188.0937, 31.916) ccw
  line L38 (-184.719, 32.844) -> (-184.0663, 30.4707)
  arc A39 (-186.392, 27.9802) -> (-184.0663, 30.4707) centre (-185.9947, 29.9403) ccw
  line L39 (-186.392, 27.9802) -> (-195.9523, 29.9181)
  arc A40 (-198.7461, 33.0725) -> (-195.9523, 29.9181) centre (-195.257, 33.3483) ccw
  arc A41 (-196.251, 35.416) -> (-198.7461, 33.0725) centre (-196.251, 32.916) ccw
  line L40 (-196.251, 35.416) -> (-188.0937, 35.416)
  line L41 (-217.2747, 25.9128) -> (-228.1983, 31.0611)
  arc A42 (-227.1325, 35.8225) -> (-228.1983, 31.0611) centre (-227.1325, 33.3225) ccw
  line L42 (-227.1325, 35.8225) -> (-210.1386, 35.8225)
  arc A43 (-208.6312, 32.5081) -> (-210.1386, 35.8225) centre (-210.1386, 33.8225) ccw
  line L43 (-208.6312, 32.5081) -> (-213.7346, 26.655)
  arc A44 (-217.2747, 25.9128) -> (-213.7346, 26.655) centre (-215.9958, 28.6265) ccw
  line L44 (-275.2388, 10.4141) -> (-270.0721, 20.3076)
  arc A45 (-266.8843, 20.7953) -> (-270.0721, 20.3076) centre (-268.2993, 19.3818) ccw
  line L45 (-266.8843, 20.7953) -> (-256.1487, 10.0484)
  arc A46 (-257.2099, 7.4883) -> (-256.1487, 10.0484) centre (-257.2099, 8.9883) ccw
  line L46 (-257.2099, 7.4883) -> (-273.466, 7.4883)
  arc A47 (-275.2388, 10.4141) -> (-273.466, 7.4883) centre (-273.466, 9.4883) ccw
  arc A48 (-241.9344, 18.6588) -> (-243.5581, 13.7607) centre (-241.2933, 15.7281) ccw
  line L47 (-241.9344, 18.6588) -> (-239.6311, 19.1626)
  arc A49 (-235.9763, 18.1116) -> (-239.6311, 19.1626) centre (-238.7763, 15.255) ccw
  line L48 (-235.9763, 18.1116) -> (-232.7955, 14.9938)
  arc A50 (-232.5294, 12.459) -> (-232.7955, 14.9938) centre (-234.1955, 13.5655) ccw
  line L49 (-232.5294, 12.459) -> (-235.3648, 8.1899)
  arc A51 (-238.5407, 7.9849) -> (-235.3648, 8.1899) centre (-237.0309, 9.2965) ccw
  line L50 (-238.5407, 7.9849) -> (-243.5581, 13.7607)
  arc A52 (-212.773, 14.8416) -> (-216.7262, 15.5987) centre (-215.2883, 12.4077) ccw
  line L51 (-212.773, 14.8416) -> (-208.1185, 10.0313)
  arc A53 (-209.1965, 7.4883) -> (-208.1185, 10.0313) centre (-209.1965, 8.9883) ccw
  line L52 (-209.1965, 7.4883) -> (-221.7705, 7.4883)
  arc A54 (-225.7961, 9.9772) -> (-221.7705, 7.4883) centre (-221.7705, 11.9883) ccw
  arc A55 (-225.0064, 11.8674) -> (-225.7961, 9.9772) centre (-224.3901, 10.4998) ccw
  line L53 (-225.0064, 11.8674) -> (-216.7262, 15.5987)
  arc A56 (-174.0246, 11.1932) -> (-171.6146, 10.8227) centre (-172.6868, 11.8717) ccw
  line L54 (-174.0246, 11.1932) -> (-181.8959, 26.7134)
  arc A57 (-182.3695, 30.8671) -> (-181.8959, 26.7134) centre (-176.5448, 29.4273) ccw
  line L55 (-182.3695, 30.8671) -> (-181.99, 32.4024)
  arc A58 (-177.6214, 35.8225) -> (-181.99, 32.4024) centre (-177.6214, 31.3225) ccw
  line L56 (-177.6214, 35.8225) -> (-151.9101, 35.8225)
  arc A59 (-150.4805, 32.4238) -> (-151.9101, 35.8225) centre (-151.9101, 33.8225) ccw
  line L57 (-150.4805, 32.4238) -> (-171.6146, 10.8227)
  line L58 (-82.205, 31.3656) -> (-72.5578, 17.4373)
  arc A60 (-72.8035, 13.7118) -> (-72.5578, 17.4373) centre (-75.024, 15.7291) ccw
  line L59 (-72.8035, 13.7118) -> (-73.5988, 12.8364)
  arc A61 (-78.0703, 11.8224) -> (-73.5988, 12.8364) centre (-76.5594, 15.5261) ccw
  line L60 (-78.0703, 11.8224) -> (-104.2986, 22.522)
  arc A62 (-105.4935, 24.8169) -> (-104.2986, 22.522) centre (-103.5432, 24.3738) ccw
  line L61 (-105.4935, 24.8169) -> (-103.8723, 31.9532)
  arc A63 (-99.4841, 35.4563) -> (-103.8723, 31.9532) centre (-99.4841, 30.9563) ccw
  line L62 (-99.4841, 35.4563) -> (-90.0147, 35.4563)
  arc A64 (-82.205, 31.3656) -> (-90.0147, 35.4563) centre (-90.0147, 25.9563) ccw
  line L63 (-33.0847, 15.2132) -> (-33.932, 14.2042)
  arc A65 (-37.8488, 14.315) -> (-33.932, 14.2042) centre (-35.8465, 15.812) ccw
  line L64 (-37.8488, 14.315) -> (-50.0683, 30.66)
  arc A66 (-47.6655, 35.4563) -> (-50.0683, 30.66) centre (-47.6655, 32.4563) ccw
  line L65 (-47.6655, 35.4563) -> (-19.3029, 35.4563)
  arc A67 (-18.1542, 32.9917) -> (-19.3029, 35.4563) centre (-19.3029, 33.9563) ccw
  line L66 (-18.1542, 32.9917) -> (-20.1473, 30.6184)
  line L67 (-20.1473, 30.6184) -> (-29.0847, 30.6184)
  arc A68 (-29.0847, 30.6184) -> (-33.0847, 26.6184) centre (-29.0847, 26.6184) ccw
  line L68 (-33.0847, 26.6184) -> (-33.0847, 15.2132)
  line L69 (-78.6079, 35.4563) -> (-54.4585, 35.4563)
  arc A69 (-53.4418, 32.8535) -> (-54.4585, 35.4563) centre (-54.4585, 33.9563) ccw
  line L70 (-53.4418, 32.8535) -> (-67.1338, 20.2294)
  arc A70 (-72.3955, 20.8271) -> (-67.1338, 20.2294) centre (-69.5063, 22.8025) ccw
  line L71 (-72.3955, 20.8271) -> (-80.2589, 32.3275)
  arc A71 (-78.6079, 35.4563) -> (-80.2589, 32.3275) centre (-78.6079, 33.4563) ccw
  arc A72 (-130.3627, 33.6384) -> (-133.2496, 35.8225) centre (-133.2496, 32.8225) ccw
  line L72 (-130.3627, 33.6384) -> (-123.8711, 10.6682)
  arc A73 (-126.2769, 7.4883) -> (-123.8711, 10.6682) centre (-126.2769, 9.9883) ccw
  line L73 (-126.2769, 7.4883) -> (-169.5459, 7.4883)
  arc A74 (-170.2607, 9.1876) -> (-169.5459, 7.4883) centre (-169.5459, 8.4883) ccw
  line L74 (-170.2607, 9.1876) -> (-147.4375, 32.5152)
  arc A75 (-139.5747, 35.8225) -> (-147.4375, 32.5152) centre (-139.5747, 24.8225) ccw
  line L75 (-139.5747, 35.8225) -> (-133.2496, 35.8225)
  arc A76 (-204.0082, 7.8292) -> (-200.5039, 9.0318) centre (-202.5008, 9.1436) ccw
  line L76 (-204.0082, 7.8292) -> (-212.1436, 17.1592)
  arc A77 (-212.4198, 22.0615) -> (-212.1436, 17.1592) centre (-209.1287, 19.7881) ccw
  line L77 (-212.4198, 22.0615) -> (-206.287, 30.9396)
  arc A78 (-201.8048, 31.4581) -> (-206.287, 30.9396) centre (-203.8187, 29.2345) ccw
  line L78 (-201.8048, 31.4581) -> (-201.3181, 31.0173)
  arc A79 (-199.5188, 26.6333) -> (-201.3181, 31.0173) centre (-205.0102, 26.9407) ccw
  line L79 (-199.5188, 26.6333) -> (-200.5039, 9.0318)
  arc A80 (-236.0861, 22.7103) -> (-234.8254, 23.9119) centre (-236.6979, 24.6145) ccw
  line L80 (-236.0861, 22.7103) -> (-240.9685, 21.1417)
  arc A81 (-244.0157, 20.865) -> (-240.9685, 21.1417) centre (-243.1097, 27.8062) ccw
  line L81 (-244.0157, 20.865) -> (-246.7988, 21.2283)
  arc A82 (-248.9657, 21.9955) -> (-246.7988, 21.2283) centre (-246.087, 26.682) ccw
  line L82 (-248.9657, 21.9955) -> (-263.938, 31.1923)
  arc A83 (-262.6295, 35.8225) -> (-263.938, 31.1923) centre (-262.6295, 33.3225) ccw
  line L83 (-262.6295, 35.8225) -> (-234.1781, 35.8225)
  arc A84 (-233.2969, 35.2953) -> (-234.1781, 35.8225) centre (-234.1781, 34.8225) ccw
  line L84 (-233.2969, 35.2953) -> (-232.701, 34.1846)
  arc A85 (-232.4395, 30.2703) -> (-232.701, 34.1846) centre (-236.8867, 31.939) ccw
  line L85 (-232.4395, 30.2703) -> (-234.8254, 23.9119)
  arc A86 (-267.8373, 31.4338) -> (-270.4965, 35.8225) centre (-270.4965, 32.8225) ccw
  line L86 (-267.8373, 31.4338) -> (-275.7739, 16.2362)
  arc A87 (-281.8887, 15.022) -> (-275.7739, 16.2362) centre (-279.3195, 18.0878) ccw
  line L87 (-281.8887, 15.022) -> (-282.1098, 15.2072)
  arc A88 (-283.8736, 21.9137) -> (-282.1098, 15.2072) centre (-278.256, 19.8059) ccw
  line L88 (-283.8736, 21.9137) -> (-279.385, 33.8764)
  arc A89 (-276.5762, 35.8225) -> (-279.385, 33.8764) centre (-276.5762, 32.8225) ccw
  line L89 (-276.5762, 35.8225) -> (-270.4965, 35.8225)
  line L90 (-298.2923, 37.3) -> (-298, 21.0097)
  line L91 (-298, 21.0097) -> (-298.5325, 4.9975)
  line L92 (-298.5325, 4.9975) -> (-2.7182, 4.9975)
  line L93 (-2.9579, 37.3) -> (-298.2923, 37.3)
  line L94 (-28.0847, 29.6184) -> (-18.0847, 29.6184)
  line L95 (-14.0847, 25.6184) -> (-14.0847, 15.6184)
  line L96 (-18.0847, 11.6184) -> (-28.0847, 11.6184)
  line L97 (-32.0847, 15.6184) -> (-32.0847, 25.6184)
  arc A90 (-28.0847, 29.6184) -> (-32.0847, 25.6184) centre (-28.0847, 25.6184) ccw
  arc A91 (-14.0847, 25.6184) -> (-18.0847, 29.6184) centre (-18.0847, 25.6184) ccw
  arc A92 (-18.0847, 11.6184) -> (-14.0847, 15.6184) centre (-18.0847, 15.6184) ccw
  arc A93 (-32.0847, 15.6184) -> (-28.0847, 11.6184) centre (-28.0847, 15.6184) ccw
  arc A94 (-15.0847, 25.6184) -> (-18.0847, 28.6184) centre (-18.0847, 25.6184) ccw
  line L98 (-28.0847, 28.6184) -> (-18.0847, 28.6184)
  arc A95 (-28.0847, 28.6184) -> (-31.0847, 25.6184) centre (-28.0847, 25.6184) ccw
  line L99 (-31.0847, 15.6184) -> (-31.0847, 25.6184)
  arc A96 (-31.0847, 15.6184) -> (-28.0847, 12.6184) centre (-28.0847, 15.6184) ccw
  line L100 (-18.0847, 12.6184) -> (-28.0847, 12.6184)
  arc A97 (-18.0847, 12.6184) -> (-15.0847, 15.6184) centre (-18.0847, 15.6184) ccw
  line L101 (-15.0847, 25.6184) -> (-15.0847, 15.6184)
  line L102 (-2.7182, 4.9975) -> (-3.2016, 19.5338)
  line L103 (-3.1358, 27.3863) -> (-2.9579, 37.3)
  arc A98 (-3.3467, 19.0615) -> (-3.2016, 19.5338) centre (-15.2208, 22.9673) ccw
  line L104 (-3.7376, 32.7885) -> (-3.1358, 27.3863)
  arc A99 (-293.8507, 35.1983) -> (-296.4896, 32.1574) centre (-293.4902, 32.2201) ccw
  line L105 (-293.8507, 35.1983) -> (-291.141, 35.5263)
  line L106 (-295.3907, 10.7748) -> (-295.786, 17.2442)
  arc A100 (-293.5794, 18.6573) -> (-295.786, 17.2442) centre (-294.2888, 17.3357) ccw
  point P0 (-32.0847, 29.6184)
  point P1 (-14.0847, 29.6184)
  point P2 (-32.0847, 11.6184)
  dimension "d643" = 18
  dimension "d644" = 18
  dimension "d645" = 1
  dimension "d646" = 1
  dimension "d647" = 4
  dimension "d648" = 1
  constraint horizontal L94
  constraint vertical L95
  constraint horizontal L96
  constraint vertical L97
  constraint coincident P0 L94
  constraint coincident P0 L97
  constraint tangent L94 A90
  constraint tangent L97 A90
  constraint coincident P1 L94
  constraint coincident P1 L95
  constraint tangent L94 A91
  constraint tangent L95 A91
  constraint equal A90 A91
  constraint tangent L95 A92
  constraint tangent L96 A92
  constraint equal A90 A92
  constraint coincident P2 L96
  constraint coincident P2 L97
  constraint tangent L96 A93
  constraint tangent L97 A93
  constraint equal A90 A93
  measures "d643" distance of P0 P1
  measures "d644" distance of P0 P2
  measures "d645" distance of L3 L95
  measures "d646" distance of L67 L94
  measures "d647" radius of A90
extrude "Extrude14" add sketch "Sketch24" along normal blind 1 contours L94 L95 L96 L97 A90 A91 A92 A93
extrude "Extrude15" cut sketch "Sketch24" along normal up to surface contours A94 L98 A95 L99 A96 L100 A97 L101 end surface through (-109.4382, 7.3501, 19.6195) normal (-0.992191, 0, 0.12473) offset 0